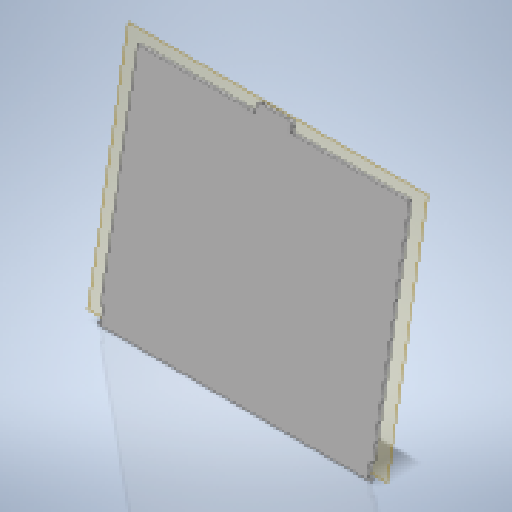
# Autodesk Inventor part: tampa
Saved by Autodesk Inventor 2024.3 (Build 283343000, 343)
## iProperties
Created: 2024-04-25
Part Number: tampa
Material: Genérico
Document SubType Name: Modeling
Designer: joaov
Density: 1 g/cm^3
Appearance: Acetinada - Limão chiffon
Author: joaov
Autodesk Inventor part; units mm, degrees
ref_plane "YZ Plane" through (0, 0, 0) normal (1, 0, 0) x (0, 1, 0)
ref_plane "XZ Plane" through (0, 0, 0) normal (0, 1, 0) x (-1, 0, 0)
ref_plane "XY Plane" through (0, 0, 0) normal (0, 0, 1) x (1, 0, 0)
ref_plane "Plano de trabalho1" through (-73.6994, 115.1379, -47.7889) normal (0.3422133, 0.1688693, 0.9243231) x (0.7308101, -0.6661496, -0.1488665)
sketch "Esboço3" plane through (-73.6994, 115.1379, -47.7889) normal (0.3422133, 0.1688693, 0.9243231) x (0.7308101, -0.6661496, -0.1488665)
  line L0 (0, 0) -> (150, 0)
  line L1 (150, 0) -> (150, 125)
  line L2 (-150, -125) -> (150, -125)
  line L3 (150, -125) -> (147, -125)
  line L4 (150, -125) -> (150, -122)
  line L5 (150, -122) -> (147, -122)
  line L6 (147, -108) -> (150, -108)
  line L7 (150, -125) -> (150, -122)
  line L8 (150, -108) -> (150, 125)
  line L9 (-150, -125) -> (-150, -122)
  line L10 (-150, -122) -> (-147, -122)
  line L11 (-147, -108) -> (-150, -108)
  line L12 (-150, 125) -> (-150, -108)
  line L13 (-150, -122) -> (-150, -125)
  line L14 (0, 135) -> (20, 135)
  line L15 (0, 135) -> (-20, 135)
  line L16 (-20, 135) -> (-20, 125)
  line L17 (20, 135) -> (20, 125)
  line L18 (150, 125) -> (20, 125)
  line L19 (-20, 125) -> (-150, 125)
  line L20 (-151, -115) -> (-151, -114)
  line L21 (-151, -114) -> (-147, -114)
  line L22 (-151, -115) -> (-151, -116)
  line L23 (-151, -116) -> (-147, -116)
  line L24 (-147, -122) -> (-147, -116)
  line L25 (-147, -114) -> (-147, -108)
  line L26 (151, -115) -> (151, -114)
  line L27 (151, -114) -> (147, -114)
  line L28 (151, -115) -> (151, -116)
  line L29 (151, -116) -> (147, -116)
  line L30 (147, -122) -> (147, -116)
  line L31 (147, -114) -> (147, -108)
  point P0 (123.4452, -56.9069)
  dimension "d24" = 150
  dimension "d25" = 125
  dimension "d26" = 300
  dimension "d27" = 250
  dimension "d33" = 3
  dimension "d34" = 3
  dimension "d37" = 20
  dimension "d43" = 1
  dimension "d44" = 1
  constraints: 64 end point, 25 perpendicular, 6 parallel, 5 horizontal, 4 vertical, 2 point on line
  measures "d24" distance of L0.start L0.end
  measures "d25" distance of L0.end L1.end
  measures "d26" distance of L2.end L2.start
  measures "d27" distance of L2.start L12.start
  measures "d33" distance of L2.start L9.end
  measures "d34" distance of L9.end L10.end
  measures "d37" distance of L14.start L14.end
  measures "d43" distance of L20.start L20.end
  measures "d44" distance of L20.start L22.end
extrude "Extrusão3" add sketch "Esboço3" along normal blind 3
fillet "Arredondamento1" radius 5 2 edges at (21.1609, 200.1388, -96.8156) (-8.0715, 226.7848, -90.8609)
sketch "Esboço4" plane through (-72.6728, 115.6445, -45.0159) normal (0.3422133, 0.1688693, 0.9243231) x (0.7308101, -0.6661496, -0.1488665)
  line L0 (150, 125) -> (20, 125) projected
  line L1 (-20, 125) -> (-150, 125) projected
  line L2 (20, 125) -> (-20, 125)
  line L3 (0, 125) -> (0, -125)
  line L4 (-150, -125) -> (150, -125) projected
  line L5 (0, 0) -> (75, 0)
  line L6 (0, 0) -> (-75, 0)
  line L7 (-75, 0) -> (-78, 0)
  line L8 (75, 0) -> (78, 0)
  circle A0 centre (78, 0) radius 3
  circle A1 centre (-78, 0) radius 3
  dimension "d48" = 75
  dimension "d49" = 75
  dimension "d50" = 3
  dimension "d51" = 3
  constraints: 12 end point, 5 horizontal, 3 midpoint, 2 coincident, 2 horizontal alignment, 4 other
  measures "d48" distance of L5.start L5.end
  measures "d49" distance of L5.start L6.end
  measures "d50" distance of L6.end L7.end
  measures "d51" distance of L5.end L8.end
extrude "Extrusão4" cut sketch "Esboço4" against normal blind 3
